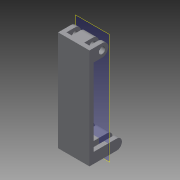
# Autodesk Inventor part: armholder
Saved by Autodesk Inventor 2015 (Build 190159000, 159)
## iProperties
Created: 2015-12-15
Part Number: armholder
Material: Generic
Document SubType Name: Modeling
Designer: Ross
Density: 1 g/cm^3
Appearance: Default
Author: Ross
Autodesk Inventor part; units mm, degrees
ref_plane "XZ Plane" through (0, 0, 0) normal (0, 1, 0) x (-1, 0, 0)
ref_plane "XY Plane" through (0, 0, 0) normal (0, 0, 1) x (1, 0, 0)
sketch "Sketch1" plane through (0, 0, 0) normal (0, 1, 0) x (-1, 0, 0)
  line L0 (0, 0) -> (15, 0)
  line L1 (15, 0) -> (15, 120)
  line L2 (15, 120) -> (0, 120)
  line L3 (0, 120) -> (0, 0)
  dimension "d0" = 15
  dimension "d1" = 120
  constraints: 8 end point, 2 parallel, 1 horizontal, 1 perpendicular
  measures "d0" distance of L2.end L1.end
  measures "d1" distance of L1.end L0.end
extrude "Extrusion1" add sketch "Sketch1" along normal blind 3
sketch "Sketch3" plane through (0, 0, 120) normal (1, 0, 0) x (0, 0, -1)
  line L0 (120, 0) -> (115, 0)
  line L1 (0, 0) -> (120, 0) projected
  line L2 (115, 0) -> (115, 3)
  line L3 (0, 3) -> (120, 3) projected
  line L4 (115, 3) -> (115, 13)
  line L5 (120, 13) -> (120, 3)
  line L6 (120, 3) -> (115, 3)
  arc A0 (120, 13) -> (115, 13) centre (117.5, 13) ccw
  dimension "d4" = 5
  dimension "d5" = 10
  constraints: 10 end point, 3 point on line, 2 perpendicular, 2 point on circle, 1 centre point
  measures "d4" distance of L0.start L0.end
  measures "d5" distance of L2.end L4.end
extrude "Extrusion2" add sketch "Sketch3" against normal blind 2
ref_plane "Work Plane1" through (-7.5, 0, 0) normal (1, 0, 0) x (0, 1, 0)
mirror "Mirror1" about plane through (-7.5, 0, 0) normal (1, 0, 0) of "Extrusion2"
ref_plane "Work Plane2" through (-4.25, 0, 0) normal (1, 0, 0) x (0, 1, 0)
mirror "Mirror2" about plane through (-4.25, 0, 0) normal (1, 0, 0) of "Extrusion2"
sketch "Sketch6" plane through (-6.5, 3, 0) normal (1, 0, 0) x (0, 0, -1)
  line L0 (0, 0) -> (-5, 0)
  line L1 (-5, 0) -> (-5, 10)
  line L2 (-5, 0) -> (-5, 10) projected
  line L3 (-5, 10) -> (-5, 0)
  arc A0 (0, 10) -> (-5, 10) centre (-2.5, 10) ccw projected
  arc A1 (0, 10) -> (-5, 10) centre (-2.5, 10) ccw
  line L4 (0, 10) -> (0, 0) projected
  line L5 (0, 10) -> (0, 0)
  point P0 (0, -3)
  constraints: 9 end point, 3 point on circle, 2 point on line, 1 centre point, 1 coincident, 1 collinear, 1 concentric, 1 horizontal, 1 tangent, 1 vertical
extrude "Extrusion3" add sketch "Sketch6" along normal blind 2
mirror "Mirror3" about plane through (-7.5, 0, 0) normal (1, 0, 0) of "Extrusion3"
sketch "Sketch9" plane through (0, 0, 120) normal (1, 0, 0) x (0, 0, -1)
  line L0 (120, 0) -> (75, 0)
  line L1 (120, 0) -> (0, 0) projected
  line L2 (75, 0) -> (75, 3)
  line L3 (0, 3) -> (115, 3) projected
  line L4 (75, 3) -> (72, 3)
  line L5 (75, 3) -> (78, 3)
  line L6 (75, 3) -> (75, 6)
  circle A0 centre (75, 6) radius 1.5
  line L7 (72, 3) -> (72, 6)
  line L8 (78, 3) -> (78, 6)
  arc A1 (78, 6) -> (72, 6) centre (75, 6) ccw
  dimension "d16" = 45
  dimension "d17" = 3
  dimension "d18" = 3
  dimension "d20" = 3
  constraints: 14 end point, 5 point on line, 2 centre point, 2 coincident, 2 point on circle, 2 vertical, 1 perpendicular
  measures "d16" distance of L0.start L0.end
  measures "d17" distance of L2.end L4.end
  measures "d18" distance of L2.end L5.end
  measures "d20" distance of L2.end L6.end
extrude "Extrusion4" add sketch "Sketch9" against normal blind 2
mirror "Mirror4" about plane through (-7.5, 0, 0) normal (1, 0, 0) of "Extrusion4"
mirror "Mirror5" about plane through (-4.25, 0, 0) normal (1, 0, 0) of "Extrusion4"
sketch "Sketch10" plane through (-6.5, 3, 42) normal (1, 0, 0) x (0, 0, -1)
  line L0 (-6, 0) -> (0, 0)
  line L1 (0, 0) -> (-6, 0) projected
  line L2 (0, 0) -> (0, 3)
  arc A0 (0, 3) -> (-6, 3) centre (-3, 3) ccw projected
  arc A1 (0, 3) -> (-6, 3) centre (-3, 3) ccw
  line L3 (-6, 0) -> (-6, 3)
  line L4 (-6, 0) -> (-6, 3) projected
  point P0 (42, -3)
  constraints: 6 end point, 2 collinear, 2 point on circle, 1 centre point, 1 coincident, 1 perpendicular, 1 tangent
extrude "Extrusion5" add sketch "Sketch10" along normal blind 2
sketch "Sketch11" plane through (-6.5, 6, 45) normal (-1, 0, 0) x (0, 0, 1)
  circle A0 centre (0, 0) radius 1.5
  point P0 (-45, -6)
  constraints: 1 centre point
extrude "Extrusion6" cut sketch "Sketch11" against normal blind 2
mirror "Mirror6" about plane through (-7.5, 0, 0) normal (1, 0, 0) of "Extrusion5", "Extrusion6"
sketch "Sketch12" plane through (0, 3, 0) normal (0, 1, 0) x (1, 0, 0)
  line L0 (0, -120) -> (-15, -120)
  line L1 (-15, -120) -> (-15, -48)
  line L2 (-15, -48) -> (0, -48)
  line L3 (0, -48) -> (0, -120)
  point P0 (0, 0)
  constraints: 8 end point, 2 parallel, 1 horizontal, 1 perpendicular
extrude "Extrusion7" cut sketch "Sketch12" against normal blind 3
sketch "Sketch13" plane through (0, 3, 0) normal (0, 1, 0) x (1, 0, 0)
  line L0 (-15, -5) -> (-15, -42)
  line L1 (-15, -42) -> (-13, -42)
  line L2 (-15, -42) -> (-13, -42) projected
  line L3 (-13, -42) -> (-13, -48)
  line L4 (-13, -42) -> (-13, -48) projected
  line L5 (-13, -48) -> (-10.5, -48)
  line L6 (-10.5, -48) -> (-10.5, -42)
  line L7 (-10.5, -48) -> (-10.5, -42) projected
  line L8 (-10.5, -42) -> (-4.5, -42)
  line L9 (-10.5, -42) -> (-4.5, -42) projected
  line L10 (-4.5, -42) -> (-4.5, -48)
  line L11 (-4.5, -48) -> (-2, -48)
  line L12 (-4.5, -48) -> (-2, -48) projected
  line L13 (-2, -48) -> (-2, -42)
  line L14 (-2, -48) -> (-2, -42) projected
  line L15 (-2, -42) -> (0, -42)
  line L16 (0, -42) -> (0, -5)
  line L17 (0, -5) -> (-2, -5)
  line L18 (-2, -5) -> (-2, 0)
  line L19 (-2, 0) -> (-4.5, 0)
  line L20 (-4.5, 0) -> (-4.5, -5)
  line L21 (-4.5, -5) -> (-10.5, -5)
  line L22 (-4.5, -5) -> (-10.5, -5) projected
  line L23 (-10.5, -5) -> (-10.5, 0)
  line L24 (-10.5, 0) -> (-13, 0)
  line L25 (-10.5, 0) -> (-13, 0) projected
  line L26 (-13, 0) -> (-13, -5)
  line L27 (-13, -5) -> (-15, -5)
  line L28 (-13, -5) -> (-15, -5) projected
  line L29 (-15, -5) -> (-15, -42)
  line L30 (-15, 0) -> (-15, -48) projected
  point P0 (0, 0)
  constraints: 42 end point, 10 collinear, 9 perpendicular, 1 point on line, 1 vertical
extrude "Extrusion8" cut sketch "Sketch13" against normal blind 1
ref_plane "Work Plane3" through (0, 9, 0) normal (0, 1, 0) x (1, 0, 0)
sketch "Sketch15" plane through (0, 9, 0) normal (0, 1, 0) x (1, 0, 0)
  line L0 (-4.5, -48) -> (-4.5, -42) projected
  line L1 (-4.5, -45) -> (-10.5, -45)
  line L2 (-10.5, -48) -> (-10.5, -42) projected
  circle A0 centre (-7.5, -45) radius 0.8
  point P0 (0, 0)
  dimension "d32" = 1.6
  constraints: 3 midpoint, 2 end point, 1 centre point
  measures "d32" diameter of A0
extrude "Extrusion9" cut sketch "Sketch15" against normal blind 3
body "Solid1"
